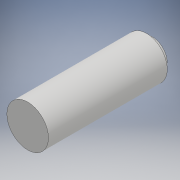
# Autodesk Inventor part: HeadScrewWithoutNot
Saved by Autodesk Inventor 2017 (Build 210142000, 142)
## iProperties
Created: 2016-12-12
Part Number: HeadScrewWithoutNot
Material: Generic
Document SubType Name: Modeling
Designer: umr
Density: 1 g/cm^3
Appearance: Default
Author: umr
Autodesk Inventor part; units mm, degrees
ref_plane "YZ Plane" through (0, 0, 0) normal (1, 0, 0) x (0, 1, 0)
ref_plane "XZ Plane" through (0, 0, 0) normal (0, 1, 0) x (-1, 0, 0)
ref_plane "XY Plane" through (0, 0, 0) normal (0, 0, 1) x (1, 0, 0)
sketch "Sketch1" plane through (0, 0, 0) normal (0, 1, 0) x (-1, 0, 0)
  circle A0 centre (0, 0) radius 2.5
  dimension "d0" = 5
  constraints: 1 centre point, 1 coincident
  measures "d0" diameter of A0
extrude "Extrusion1" add sketch "Sketch1" along normal blind 15
chamfer "Chamfer1" distance 0.7 angle 45 1 edges at (2.5, 15, 0)
body "Solid1"
